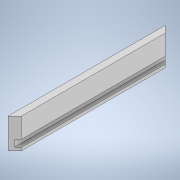
# Autodesk Inventor part: long PDMS Chamber side
Saved by Autodesk Inventor 2022 (Build 260153000, 153)
## iProperties
Created: 2022-04-27
Part Number: long PDMS Chamber side
Material: Generic
Document SubType Name: Modeling
Designer: sw_yw
Density: 1 g/cm^3
Appearance: Default
Author: sw_yw
Autodesk Inventor part; units mm, degrees
ref_plane "YZ Plane" through (0, 0, 0) normal (1, 0, 0) x (0, 1, 0)
ref_plane "XZ Plane" through (0, 0, 0) normal (0, 1, 0) x (-1, 0, 0)
ref_plane "XY Plane" through (0, 0, 0) normal (0, 0, 1) x (1, 0, 0)
sketch "Sketch1" plane through (0, 0, 0) normal (0, 1, 0) x (-1, 0, 0)
  line L0 (0, 47) -> (0, -47)
  line L1 (-4, 43) -> (-4, -43)
  line L2 (0, 0) -> (-19.6483, 0) construction
  line L3 (-4, 43) -> (0, 47)
  line L4 (0, -47) -> (-4, -43)
  point P0 (-4, 0)
  dimension "d6" = 94
  dimension "d7" = 86
  dimension "d8" = 4
  constraints: 10 end point, 2 midpoint, 2 vertical, 1 coincident, 1 horizontal, 1 point on line
  measures "d6" distance of L0.start L0.end
  measures "d7" distance of L1.start L1.end
  measures "d8" distance between parallel lines of L1 L0
extrude "Extrusion1" add sketch "Sketch1" along normal blind 18
sketch "Sketch2" plane through (4, 0, 43) normal (1, 0, 0) x (0, 0, -1)
  line L0 (-4, 0) -> (-4, 18) projected
  line L1 (90, 0) -> (90, 18) projected
  line L2 (-4, 6) -> (90, 6)
  line L3 (90, 6) -> (90, 1.9)
  line L4 (90, 1.9) -> (-4, 1.9)
  line L5 (-4, 1.9) -> (-4, 6)
  line L6 (0, 0) -> (86, 0) projected
  point P0 (43, 0)
  point P1 (-4, 1.9)
  dimension "d11" = 4.1
  dimension "d12" = 1.9
  constraints: 8 end point, 2 parallel, 2 point on line, 1 horizontal, 1 perpendicular
  measures "d11" distance of L2.end L3.end
  measures "d12" distance between parallel lines of L6 L4
extrude "Extrusion2" cut sketch "Sketch2" against normal blind 2
body "Solid1"
